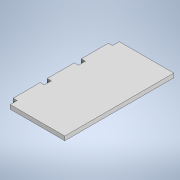
# Autodesk Inventor part: Part2
Saved by Autodesk Inventor 2022 (Build 260153000, 153)
## iProperties
Created: 2021-10-21
Part Number: Part2
Material: Generic
Document SubType Name: Modeling
Designer: Administrador
Density: 1 g/cm^3
Appearance: Default
Author: Administrador
Autodesk Inventor part; units mm, degrees
ref_plane "YZ Plane" through (0, 0, 0) normal (1, 0, 0) x (0, 1, 0)
ref_plane "XZ Plane" through (0, 0, 0) normal (0, 1, 0) x (-1, 0, 0)
ref_plane "XY Plane" through (0, 0, 0) normal (0, 0, 1) x (1, 0, 0)
sketch "Sketch1" plane through (0, 0, 0) normal (0, 1, 0) x (-1, 0, 0)
  line L0 (0, 0) -> (-40, 0)
  line L1 (-40, 0) -> (-40, -80)
  line L2 (-40, -80) -> (0, -80)
  line L3 (0, 0) -> (0, -5)
  line L4 (0, -5) -> (3, -5)
  line L5 (3, -5) -> (3, -25)
  line L6 (3, -25) -> (0, -25)
  line L7 (0, -80) -> (0, -75)
  line L8 (0, -75) -> (3, -75)
  line L9 (3, -75) -> (3, -55)
  line L10 (3, -55) -> (0, -55)
  line L11 (0, -25) -> (0, -30)
  line L12 (0, -30) -> (3, -30)
  line L13 (3, -30) -> (3, -50)
  line L14 (3, -50) -> (0, -50)
  line L15 (0, -50) -> (0, -55)
  dimension "d0" = 40
  dimension "d1" = 80
  dimension "d2" = 5
  dimension "d3" = 3
  dimension "d4" = 20
  dimension "d5" = 5
  dimension "d6" = 20
  dimension "d7" = 5
  dimension "d8" = 20
  constraints: 32 end point, 4 horizontal, 4 parallel, 4 perpendicular, 1 vertical
  measures "d0" distance of L2.end L1.end
  measures "d1" distance of L1.end L0.end
  measures "d2" distance of L0.start L3.end
  measures "d3" distance of L5.end L6.end
  measures "d4" distance of L4.end L5.end
  measures "d5" distance of L2.end L7.end
  measures "d6" distance of L9.end L8.end
  measures "d7" distance of L6.end L11.end
  measures "d8" distance of L12.end L13.end
extrude "Extrusion1" add sketch "Sketch1" along normal blind 3
body "Solid1"
